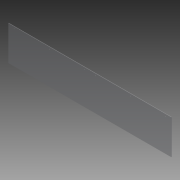
# Autodesk Inventor part: GE-13035
Saved by Autodesk Inventor 2013 (Build 170138000, 138)
## iProperties
Created: 2013-01-03
Part Number: GE-13035
Material: Polycarbonate, Clear
Document SubType Name: Modeling
Designer: Phillip
Density: 1 g/cm^3
Author: Phillip
Autodesk Inventor part; units mm, degrees
ref_plane "YZ Plane" through (0, 0, 0) normal (1, 0, 0) x (0, 1, 0)
ref_plane "XZ Plane" through (0, 0, 0) normal (0, 1, 0) x (-1, 0, 0)
ref_plane "XY Plane" through (0, 0, 0) normal (0, 0, 1) x (1, 0, 0)
sketch "Sketch1" plane through (0, 0, 0) normal (0, 0, 1) x (1, 0, 0)
  line L0 (0, 0) -> (2184.4, 0)
  line L1 (2184.4, 0) -> (2184.4, 463.55)
  line L2 (2184.4, 463.55) -> (0, 463.55)
  line L3 (0, 463.55) -> (0, 0)
  dimension "d0" = 2184.4
  dimension "d1" = 463.55
  constraints: 8 end point, 2 parallel, 1 horizontal, 1 perpendicular
  measures "d0" distance of L2.end L1.end
  measures "d1" distance of L1.end L0.end
extrude "Extrusion1" add sketch "Sketch1" against normal blind 6.35
sketch "Sketch2" plane through (0, 0, 0) normal (0, 0, 1) x (1, 0, 0)
  line L0 (2184.4, 463.55) -> (0, 463.55) projected
  line L1 (0, 463.55) -> (0, 0) projected
  point P0 (76.2, 438.15)
  point P1 (546.1, 438.15)
  point P2 (1016, 438.15)
  point P3 (1168.4, 438.15)
  point P4 (1638.3, 438.15)
  point P5 (2108.2, 438.15)
  dimension "d4" = 76.2
  dimension "d5" = 25.4
  dimension "d6" = 546.1
  dimension "d7" = 1016
  dimension "d8" = 1168.4
  dimension "d9" = 1638.3
  dimension "d10" = 2108.2
  constraints: 5 horizontal alignment
  measures "d4" distance from line of L1 point (76.2, 438.15)
  measures "d5" distance from line of point (76.2, 438.15) L0
  measures "d6" distance from line of point (546.1, 438.15) L1
  measures "d7" distance from line of point (1016, 438.15) L1
  measures "d8" distance from line of point (1168.4, 438.15) L1
  measures "d9" distance from line of point (1638.3, 438.15) L1
  measures "d10" distance from line of point (2108.2, 438.15) L1
hole "Hole1" at (76.2, 438.15, 0) at (546.1, 438.15, 0) at (1016, 438.15, 0) at (1168.4, 438.15, 0) at (1638.3, 438.15, 0) at (2108.2, 438.15, 0) direction (0, 0, -1) diameter 9.652 end through all
body "Solid1"
